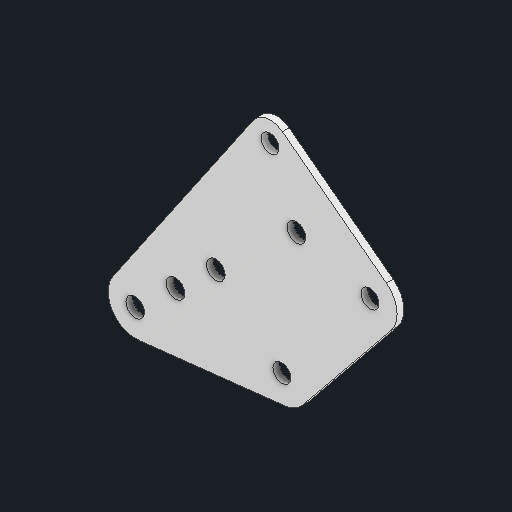
# Autodesk Inventor part: Gearbox
Saved by Autodesk Inventor 2025 (Build 290162000, 162)
## iProperties
Created: 2024-12-30
Part Number: Gearbox
Material: Acetal Resin, White
Document SubType Name: Modeling
Designer: Averey Ku
Density: 1.425 g/cm^3
Appearance: Smooth - White
Author: Averey Ku
Autodesk Inventor part; units mm, degrees
ref_plane "YZ Plane" through (0, 0, 0) normal (1, 0, 0) x (0, 1, 0)
ref_plane "XZ Plane" through (0, 0, 0) normal (0, 1, 0) x (-1, 0, 0)
ref_plane "XY Plane" through (0, 0, 0) normal (0, 0, 1) x (1, 0, 0)
sketch "main" plane through (0, 0, 0) normal (0, 0, 1) x (1, 0, 0)
  circle A0 centre (2.6045, 11.9092) radius 2.1844
  circle A1 centre (-3.5552, 26.8777) radius 2.0955
  arc A2 (-0.6729, 30.669) -> (-7.4873, 29.5648) centre (-3.5552, 26.8777) ccw
  circle A3 centre (19.8371, 7.1) radius 2.0955
  arc A4 (24.7659, 3.0962) -> (23.6801, 12.155) centre (19.8371, 7.1) ccw
  circle A5 centre (-16.2552, -5.1047) radius 2.1844
  circle A6 centre (-0.7959, -18.3) radius 2.0955
  arc A7 (-0.0936, -24.6111) -> (4.1329, -22.3038) centre (-0.7959, -18.3) ccw
  circle A8 centre (-25.6851, -13.6116) radius 2.1844
  line L0 (-34.4127, -28.4296) -> (-0.0936, -24.6111)
  circle A9 centre (-35.1149, -22.1186) radius 2.1844
  arc A10 (-40.3577, -18.5358) -> (-34.4127, -28.4296) centre (-35.1149, -22.1186) ccw
  line L1 (-7.4873, 29.5648) -> (-40.3577, -18.5358)
  line L2 (24.7659, 3.0962) -> (4.1329, -22.3038)
  line L3 (-0.6729, 30.669) -> (23.6801, 12.155)
  point P0 (-5.4325, -4.0149)
  point P1 (-6.8254, 3.4022)
  dimension "d2" = 4.191
  dimension "d3" = 12.7
  dimension "d5" = 12.7
  dimension "d6" = 12.7
  dimension "d8" = 4.191
  dimension "d9" = 9.525
  dimension "d10" = 4.191
  measures "d2" diameter of A3
  measures "d3" diameter of A4
  measures "d5" diameter of A7
  measures "d6" diameter of A10
  measures "d8" diameter of A6
  measures "d9" diameter of A2
  measures "d10" diameter of A1
sketch "Sketch1" plane through (0, 0, 0) normal (0, 0, 1) x (1, 0, 0)
  circle A0 centre (2.6045, 11.9092) radius 2.1844
  circle A1 centre (-3.5552, 26.8777) radius 2.0955
  arc A2 (-0.6729, 30.669) -> (-7.4873, 29.5648) centre (-3.5552, 26.8777) ccw
  circle A3 centre (19.8371, 7.1) radius 2.0955
  arc A4 (24.7659, 3.0962) -> (23.6801, 12.155) centre (19.8371, 7.1) ccw
  circle A5 centre (-16.2552, -5.1047) radius 2.1844
  circle A6 centre (-0.7959, -18.3) radius 2.0955
  arc A7 (-0.0936, -24.6111) -> (4.1329, -22.3038) centre (-0.7959, -18.3) ccw
  circle A8 centre (-25.6851, -13.6116) radius 2.1844
  line L0 (-34.4127, -28.4296) -> (-0.0936, -24.6111)
  circle A9 centre (-35.1149, -22.1186) radius 2.1844
  arc A10 (-40.3577, -18.5358) -> (-34.4127, -28.4296) centre (-35.1149, -22.1186) ccw
  line L1 (-7.4873, 29.5648) -> (-40.3577, -18.5358)
  line L2 (24.7659, 3.0962) -> (4.1329, -22.3038)
  line L3 (-0.6729, 30.669) -> (23.6801, 12.155)
  point P0 (0, 0)
extrude "Extrusion1" add sketch "Sketch1" along normal blind 1.5875
body "Solid1"
